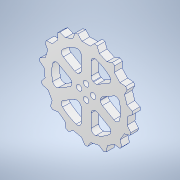
# Autodesk Inventor part: Wheel
Saved by Autodesk Inventor 2022 (Build 260153000, 153)
## iProperties
Created: 2022-08-10
Part Number: Wheel
Material: Aluminum 6061
Document SubType Name: Sheet Metal
Designer: Nick
Density: 2.7 g/cm^3
Appearance: Aluminum - Flat
Mass: 44.2813 g
Surface Area: 94.1141 cm^2
Volume: 16.4005 cm^3
Flat Pattern Width: 7.59914 cm
Flat Pattern Length: 7.5593 cm
Flat Pattern Area: 57.4442 cm^2
Sheet Metal Rule: Default
Sheet Metal Width: 2.992 in
Sheet Metal Length: 2.976 in
Sheet Metal Area: 8.904 in^2
Author: Nick
Autodesk Inventor part; units mm, degrees
ref_plane "YZ Plane" through (0, 0, 0) normal (1, 0, 0) x (0, 1, 0)
ref_plane "XZ Plane" through (0, 0, 0) normal (0, 1, 0) x (-1, 0, 0)
ref_plane "XY Plane" through (0, 0, 0) normal (0, 0, 1) x (1, 0, 0)
sketch "Sketch5" plane through (0, 0, 0) normal (0, 0, 1) x (1, 0, 0)
  circle A0 centre (0, 0) radius 38.1
  line L0 (-6.7736, 37.493) -> (-3.3806, 34.1)
  line L1 (-3.3806, 34.1) -> (3.3806, 34.1)
  line L2 (3.3806, 34.1) -> (6.7736, 37.493)
  circle A1 centre (0, 0) radius 5.75
  dimension "d20" = 76.2
  dimension "d21" = 11.5
  dimension "d22" = 4
  dimension "d23" = 135
  dimension "d24" = 135
  constraints: 6 end point, 2 centre point, 2 coincident, 2 point on circle, 1 horizontal, 1 perpendicular
  measures "d20" diameter of A0
  measures "d21" diameter of A1
  measures "d22" distance edge to line of A0 L1
  measures "d23" angle of L2 L1
  measures "d24" angle of L0 L1
extrude "Extrusion4" add sketch "Sketch5" along normal blind 6.35 contours A0 L0 L1 L2 | L2 L1 L0 A0 | A1
extrude "Extrusion5" cut sketch "Sketch5" along normal blind 6.35 contours L2 L1 L0 A0 picked at (0.7562, 35.4108)
pattern_circular "Circular Pattern2" count 15 over 360 about axis through (0, 0, 0) along (0, 0, 1) of "Extrusion5"
sketch "Sketch6" plane through (0, 0, 6.35) normal (0, 0, 1) x (1, 0, 0)
  circle A0 centre (0, 0) radius 28.1
  circle A1 centre (0, 0) radius 11.75
  line L0 (-3.4069, 28.1) -> (3.4069, 28.1) construction
  line L1 (3.3806, 34.1) -> (-3.3806, 34.1) construction
  line L2 (0, 0) -> (0, 8) construction
  circle A2 centre (0, 0) radius 5.75 projected
  line L3 (-4, 11.0482) -> (-4, 27.8138)
  line L4 (4, 27.8138) -> (4, 11.0482)
  line L5 (7.568, 8.9882) -> (22.0875, 17.371)
  line L6 (0, 0) -> (13.6183, 7.8626)
  point P0 (0, 28.1)
  dimension "d34" = 6
  dimension "d43" = 6
  dimension "d57" = 4
  dimension "d58" = 4
  dimension "d59" = 60
  dimension "d60" = 4
  dimension "d61" = 8
  constraints: 12 end point, 6 point on circle, 3 coincident, 2 centre point, 2 vertical, 2 vertical alignment, 1 horizontal, 1 midpoint, 1 parallel, 1 tangent
  measures "d34" distance between parallel lines of L0 L1
  measures "d57" distance between parallel lines of L4 L2
  measures "d58" distance between parallel lines of L3 L2
  measures "d59" angle of L6 L2
  measures "d60" distance between parallel lines of L6 L5
  measures "d61" distance between parallel lines of L4 L3
extrude "Extrusion6" cut sketch "Sketch6" against normal blind 25.4 contours L5 A1 L4 A0
fillet "Fillet1" radius 3.175 4 edges at (4, 11.0482, 3.175) (7.568, 8.9882, 3.175) (22.0875, 17.371, 3.175) (4, 27.8138, 3.175)
pattern_circular "Circular Pattern3" count 6 over 360 about axis through (0, 0, 0) along (0, 0, 1) of "Extrusion6", "Fillet1"
sketch "Sketch7" plane through (0, 0, 6.35) normal (0, 0, 1) x (1, 0, 0)
  circle A0 centre (0, 0) radius 5.75 projected
  point P0 (0, 5.75)
  constraints: 2 vertical alignment, 1 other
hole "Hole1" at (0, 5.75, 6.35) direction (0, 0, -1) diameter 4.4958 depth 14.1986 tip angle 118 clearance for "Flat Head Machine Screw" size "M4" standard "Ansi Metric M Profile"
pattern_circular "Circular Pattern4" count 4 over 360 about axis through (0, 0, 6.35) along (0, 0, -1) of "Hole1"
equation "\"d58\" = d57"
equation "\"d60\" = d57"
equation "\"BendRadius\" = Thickness"
equation "\"BendReliefWidth\" = Thickness"
equation "\"BendReliefDepth\" = 0.5 * Thickness"
equation "\"CornerReliefSize\" = 4 * Thickness"
equation "\"MinimumRemnant\" = 2 * Thickness"
equation "\"TransitionRadius\" = BendRadius"
equation "\"JacobiRadiusSize\" = BendRadius"
equation "\"GapSize\" = Thickness"
equation "\"Thickness\" = 6.35"
body "Solid2"
